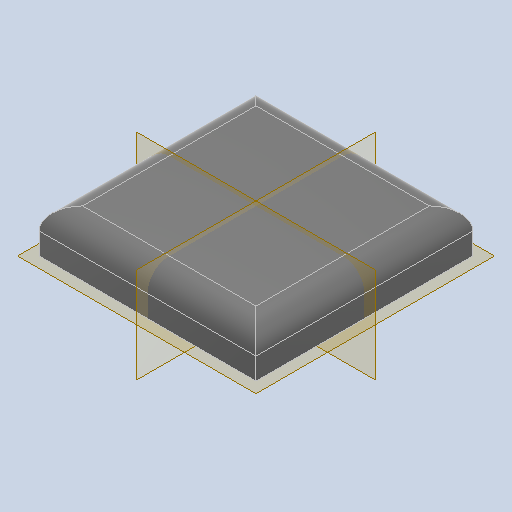
# Autodesk Inventor part: TAMPA_001_001
Saved by Autodesk Inventor 2026 (Build 300175000, 175)
## iProperties
Created: 2025-05-23
Part Number: TAMPA_001_001
Material: Rubber, Silicone
Document SubType Name: Modeling
Designer: carlo
Density: 1.25 g/cm^3
Appearance: Smooth - Black
Description: 20x20
Author: carlo
## iProperties of the stored document tampa_001_001_3DPrint.ipt
Created: 2025-05-27
Part Number: tampa_001_001_3DPrint
Material: Generic
Document SubType Name: Modeling
Designer: Carlos Dias
Density: 1 g/cm^3
Appearance: Default
Author: Carlos Dias
Autodesk Inventor part; units mm, degrees
sketch "Sketch1" plane through (0, 0, 0) normal (0, 1, 0) x (-1, 0, 0)
  line L0 (-10, 10) -> (10, 10)
  line L1 (10, 10) -> (10, -10)
  line L2 (10, -10) -> (-10, -10)
  line L3 (-10, -10) -> (-10, 10)
  line L4 (-10, 10) -> (10, -10) construction
  line L5 (10, 10) -> (-10, -10) construction
  circle A0 centre (0, 0) radius 2.4
  dimension "d0" = 20
  dimension "d3" = 4.8
  constraints: 12 end point, 2 midpoint, 2 parallel, 2 perpendicular, 1 centre point, 1 coincident, 1 horizontal
  measures "d0" distance of L1.end L2.end
  measures "d3" diameter of A0
extrude "Extrusion1" add sketch "Sketch1" along normal mid plane 8 contours A0
extrude "Extrusion2" add sketch "Sketch1" along normal blind 4
fillet "Fillet1" radius 2 4 edges at (-10, 4, 0) (0, 4, -10) (10, 4, 0) (0, 4, 10)
body "Solid1"
